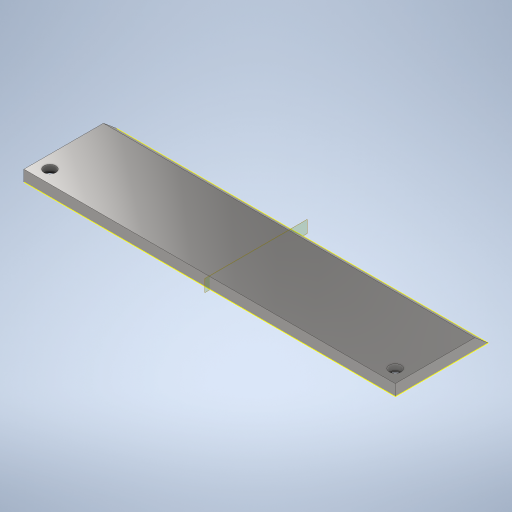
# Autodesk Inventor part: nóź
Saved by Autodesk Inventor 2023 (Build 270158000, 158)
## iProperties
Created: 2025-01-11
Part Number: nóź
Material: Stal, odlew
Document SubType Name: Modeling
Designer: kamil
Density: 7.85 g/cm^3
Appearance: Częściowo polerowany
Mass: 54.0865 g
Surface Area: 55.6523 cm^2
Volume: 6.89 cm^3
Author: kamil
Autodesk Inventor part; units mm, degrees
ref_plane "YZ Plane" through (0, 0, 0) normal (1, 0, 0) x (0, 1, 0)
ref_plane "XZ Plane" through (0, 0, 0) normal (0, 1, 0) x (-1, 0, 0)
ref_plane "XY Plane" through (0, 0, 0) normal (0, 0, 1) x (1, 0, 0)
sketch "Szkic1" plane through (0, 0, 0) normal (0, 1, 0) x (-1, 0, 0)
  line L0 (0, 0) -> (-100, 0)
  line L1 (-100, 0) -> (-100, -25)
  line L2 (-100, -25) -> (0, -25)
  line L3 (0, -25) -> (0, 0)
  dimension "d0" = 100
  dimension "d1" = 25
  constraints: 8 end point, 2 parallel, 1 horizontal, 1 perpendicular
  measures "d0" distance of L2.end L1.end
  measures "d1" distance of L1.end L0.end
extrude "Wyciągnięcie proste1" add sketch "Szkic1" along normal blind 3
sketch "Szkic2" plane through (100, 0, 0) normal (1, 0, 0) x (0, 0, -1)
  line L0 (0, 0) -> (25, 0) projected
  line L1 (25, 0) -> (25, 3) projected
  line L2 (0, 3) -> (25, 3) projected
  line L3 (0, 0) -> (0, 3) projected
  line L4 (25, 0) -> (21.4247, 3)
  dimension "d4" = 40
  constraints: 2 end point, 1 point on line
  measures "d4" angle of L0 L4
extrude "Wyciągnięcie proste2" cut sketch "Szkic2" against normal through all contours L4 L2 L1
sketch "Szkic3" plane through (0, 0, 0) normal (0, -1, 0) x (1, 0, 0)
  line L0 (0, -25) -> (0, 0) projected
  line L1 (100, 0) -> (100, -25) projected
  line L2 (0, 0) -> (100, 0) projected
  line L3 (0, -25) -> (0, 0) projected
  line L4 (100, -25) -> (0, -25) projected
  point P0 (3.5, -3.5)
  dimension "d7" = 3.5
  dimension "d8" = 3.5
  measures "d7" distance from line of point (3.5, -3.5) L2
  measures "d8" distance from line of L0 point (3.5, -3.5)
hole "Otwór1" at (3.5, 0, -3.5) direction (0, 1, 0) diameter 3.2 end through all countersink diameter 6 countersink angle 90
ref_plane "Płaszczyzna konstrukcyjna1" through (50, 0, 0) normal (-1, 0, 0) x (0, 0, 1)
mirror "Odbij1" about plane through (50, 0, 0) normal (-1, 0, 0) of "Otwór1"
sketch "Szkic4" plane through (0, 0, 0) normal (0, -1, 0) x (1, 0, 0)
  circle A0 centre (3.5, -3.5) radius 1.6 projected
  circle A1 centre (96.5, -3.5) radius 1.6 projected
  line L0 (100, 0) -> (100, -25) projected
  line L1 (100, -25) -> (0, -25) projected
  line L2 (0, -25) -> (0, 0) projected
  line L3 (0, 0) -> (100, 0) projected
